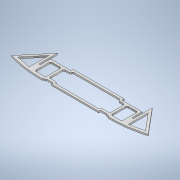
# Autodesk Inventor part: bulkhead_B1
Saved by Autodesk Inventor 2020.3 (Build 243373010, 373A)
## iProperties
Created: 2020-05-22
Part Number: bulkhead_B1
Material: Generic
Document SubType Name: Modeling
Designer: kardo
Density: 1 g/cm^3
Appearance: Default
Mass: 3.41453 g
Surface Area: 52.3935 cm^2
Volume: 3.41453 cm^3
Author: kardo
Autodesk Inventor part; units mm, degrees
ref_plane "YZ Plane" through (0, 0, 0) normal (1, 0, 0) x (0, 1, 0)
ref_plane "XZ Plane" through (0, 0, 0) normal (0, 1, 0) x (-1, 0, 0)
ref_plane "XY Plane" through (0, 0, 0) normal (0, 0, 1) x (1, 0, 0)
derived "base_sketch.ipt"
sketch "bulkhead_B1" plane through (0, -102, 0) normal (0, 1, 0) x (-1, 0, 0)
  line L0 (19.176, 46.818) -> (62.322, 46.818)
  line L1 (0, 19.935) -> (0, 0)
  line L2 (62.322, 46.818) -> (62.322, 13.529)
  line L3 (0, 5.6919) -> (-27.3644, 38.3035)
  line L4 (62.322, 44.7066) -> (19.176, 44.7066)
  line L5 (-38.352, 36.72) -> (-38.352, 34.6086) construction
  line L6 (-19.176, 42.5952) -> (-19.176, 40.4838) construction
  line L7 (0, 45.9) -> (0, 43.7886) construction
  line L8 (19.176, 46.818) -> (19.176, 44.7066) construction
  line L9 (0, 19.935) -> (28.764, 19.935)
  line L10 (28.764, 19.935) -> (28.764, 13.529)
  line L11 (28.764, 13.529) -> (62.322, 13.529)
  line L12 (62.322, 13.7901) -> (28.764, 13.7901)
  line L13 (28.764, 13.7901) -> (28.764, 16.8245)
  line L14 (28.764, 16.8245) -> (0, 16.8245)
  line L15 (0, 16.8245) -> (0, 5.6919)
  spline S0 degree 4 poles (-57.528, 27.54) (-46.0483, 34.2051) (-30.6129, 40.5281) (-11.2214, 45.0414) (8.3201, 46.818) (15.5662, 46.818) (19.176, 46.818) knots 0 0 0 0 0 0.630279 0.815816 1 1 1 1 1
  spline S1 degree 3 poles (19.176, 44.7066) (-0.1981, 44.9447) (-19.6083, 41.6917) (-38.352, 34.6086) knots 0 0 0 0 1 1 1 1
  point P0 (0, 3.825)
  point P1 (0, 13.7901)
ref_plane "bulkhead_B1_plane" through (0, -102, 0) normal (0, 1, 0) x (-1, 0, 0)
sketch "Sketch2" plane through (0, -102, 0) normal (0, 1, 0) x (-1, 0, 0)
  spline S0 degree 3 poles (19.176, 44.7066) (-0.1981, 44.9447) (-19.6083, 41.6917) (-38.352, 34.6086) knots 0 0 0 0 1 1 1 1 projected
  line L0 (62.322, 44.7066) -> (19.176, 44.7066) projected
  line L1 (62.322, 46.818) -> (62.322, 13.529) projected
  line L2 (0, 5.6919) -> (-27.3644, 38.3035) projected
  line L3 (0, 16.8245) -> (0, 3.825) projected
  line L4 (28.764, 16.8245) -> (0, 16.8245) projected
  line L5 (28.764, 13.7901) -> (28.764, 16.8245) projected
  line L6 (62.322, 13.7901) -> (28.764, 13.7901) projected
  line L7 (-21.8143, 36.3564) -> (-3, 13.9343)
  line L8 (-3, 13.9343) -> (-3, 40.1276)
  line L9 (-3, 40.1276) -> (-21.8143, 36.3564)
  line L10 (5, 38.7886) -> (5, 21.8245)
  line L11 (7, 19.8245) -> (17.176, 19.8245)
  line L12 (19.176, 21.8245) -> (19.176, 38.7886)
  line L13 (17.176, 40.7886) -> (7, 40.7886)
  line L14 (22.176, 37.3066) -> (22.176, 21.8245)
  line L15 (32.6089, 16.7901) -> (62.322, 16.7901)
  line L16 (62.322, 41.7066) -> (34.0605, 41.7066)
  line L17 (0, 16.8245) -> (0, 30.3066)
  line L18 (-27.3644, 38.3035) -> (0, 43.7886) construction
  arc A0 (19.176, 38.7886) -> (17.176, 40.7886) centre (17.176, 38.7886) ccw
  arc A1 (7, 40.7886) -> (5, 38.7886) centre (7, 38.7886) ccw
  arc A2 (5, 21.8245) -> (7, 19.8245) centre (7, 21.8245) ccw
  arc A3 (17.176, 19.8245) -> (19.176, 21.8245) centre (17.176, 21.8245) ccw
  arc A4 (24.176, 39.3066) -> (22.176, 37.3066) centre (24.176, 37.3066) ccw
  line L19 (0, 30.3066) -> (0, 43.7886) construction
  line L20 (0, 30.3066) -> (2, 30.3066)
  line L21 (2, 30.3066) -> (2, 16.6552)
  line L22 (19.176, 44.7066) -> (19.176, 43.5066)
  line L23 (19.176, 43.5066) -> (22.176, 43.5066)
  line L24 (25.176, 43.5066) -> (25.176, 44.7066) construction
  line L25 (22.176, 43.5066) -> (22.176, 42.3066)
  line L26 (22.176, 42.3066) -> (31.176, 42.3066)
  line L27 (31.176, 42.3066) -> (31.176, 44.7066)
  line L28 (22.176, 21.8245) -> (22.176, 19.8245) construction
  line L29 (22.176, 19.8245) -> (24.1745, 19.7471) construction
  line L30 (24.1745, 19.7471) -> (29.3424, 19.5471)
  line L31 (29.3424, 19.5471) -> (30.3415, 19.5085) construction
  line L32 (30.3415, 19.5085) -> (30.764, 18.6023) construction
  spline S1 degree 3 poles (22.176, 21.8245) (22.176, 20.7294) (23.0802, 19.7895) (24.1745, 19.7471) knots 0 0 0 0 1 1 1 1
  spline S2 degree 3 poles (29.3424, 19.5471) (29.9526, 19.5235) (30.5059, 19.1557) (30.764, 18.6023) knots 0 0 0 0 1 1 1 1
  line L33 (30.764, 18.6023) -> (31.1865, 17.6962)
  line L34 (31.1865, 17.6962) -> (31.6091, 16.7901) construction
  line L35 (31.6091, 16.7901) -> (32.6089, 16.7901) construction
  spline S3 degree 3 poles (31.1865, 17.6962) (31.4427, 17.1468) (32.0027, 16.7901) (32.6089, 16.7901) knots 0 0 0 0 1 1 1 1
  line L36 (31.176, 39.3066) -> (24.176, 39.3066)
  line L37 (31.176, 39.3066) -> (32.0587, 39.3066) construction
  line L38 (32.0587, 39.3066) -> (32.4317, 40.1066) construction
  line L39 (32.4317, 40.1066) -> (32.8048, 40.9066)
  line L40 (32.8048, 40.9066) -> (33.1778, 41.7066) construction
  line L41 (33.1778, 41.7066) -> (34.0605, 41.7066) construction
  spline S4 degree 3 poles (31.176, 39.3066) (31.7112, 39.3066) (32.2056, 39.6216) (32.4317, 40.1066) knots 0 0 0 0 1 1 1 1
  spline S5 degree 3 poles (32.8048, 40.9066) (33.031, 41.3917) (33.5254, 41.7066) (34.0605, 41.7066) knots 0 0 0 0 1 1 1 1
  line L42 (22.176, 43.5066) -> (25.176, 43.5066) construction
  point P0 (0, 0)
  point P1 (5, 40.7886)
  point P2 (2, 16.8245)
  point P3 (26.7584, 19.6471)
  dimension "d1" = 3
  dimension "d2" = 3
  dimension "d4" = 3
  dimension "d6" = 3
  dimension "d9" = 3
  dimension "d11" = 3
  dimension "d13" = 3
  dimension "d14" = 2
  dimension "d20" = 3
  dimension "d21" = 2
  dimension "d22" = 1.2
  dimension "d23" = 1.2
  dimension "d24" = 6
  dimension "d25" = 6
  dimension "d26" = 3
  dimension "d28" = 0.2
  dimension "d29" = 2
  dimension "d33" = 5
  dimension "d34" = 115
  dimension "d35" = 2
  dimension "d36" = 2
  dimension "d37" = 115
  dimension "d38" = 3
  constraints: 72 end point, 14 parallel, 11 equal length, 10 collinear, 10 point on circle, 10 tangent, 9 point on line, 5 centre point, 5 perpendicular, 4 horizontal, 3 equal radius, 1 midpoint, 1 vertical, 19 other
  measures "d2" distance between parallel lines of L3 L8
  measures "d4" distance between parallel lines of L4 L11
  measures "d6" vertical distance of point (5, 40.789) L18.end
  measures "d9" distance between parallel lines of L0 L16
  measures "d11" distance between parallel lines of L6 L15
  measures "d13" distance between parallel lines of L18 L9
  measures "d14" radius of A0
  measures "d20" distance between parallel lines of L10 L21
  measures "d21" distance between parallel lines of L21 L17
  measures "d22" distance of L0.end L22.end
  measures "d23" distance of L23.end L25.end
  measures "d24" distance of L22.end L24.start
  measures "d25" distance between parallel lines of L27 L24
  measures "d26" distance between parallel lines of L14 L12
  measures "d28" vertical distance of L29.end L30.end
  measures "d29" radius of A4
  measures "d33" distance from line of L4 L14.end
  measures "d34" angle of L15 L33
  measures "d35" distance of L14.end L28.end
  measures "d36" distance from line of L5 L32.end
  measures "d37" angle of L36 L39
  measures "d38" distance between parallel lines of L26 L36
extrude "Extrusion1" add sketch "Sketch2" along normal blind 2 contours L22 L23 L25 L26 L27 L0 L1 L16 S5 L39 S4 L36 A4 L14 S1 L30 S2 L33 S3 L15 L6 L5 L4 L21 L20 L17 L3 L2 S0
mirror "Mirror1" about plane through (-62.322, -102, 13.7901) normal (-1, 0, 0) of "Extrusion1"
equation "\"d21\" = stringer_thickness"
equation "\"d22\" = decking_thickness"
equation "\"d23\" = decking_thickness"
equation "\"d24\" = cowl_strip_width"
equation "\"d25\" = cowl_insulation_width"
equation "\"d18\" = bulkhead_thickness"
equation "\"stringer_thickness\" = 2"
equation "\"decking_thickness\" = 1.2"
equation "\"cowl_strip_width\" = 6"
equation "\"cowl_insulation_width\" = 6"
equation "\"bulkhead_thickness\" = 2"
body "Solid1"
